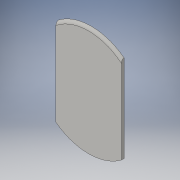
# Autodesk Inventor part: Nathan_RobotArm_Base
Saved by Autodesk Inventor 2016 (Build 200138000, 138)
## iProperties
Created: 2017-03-30
Part Number: Nathan_RobotArm_Base
Material: Generic
Document SubType Name: Modeling
Designer: brandn
Density: 1 g/cm^3
Appearance: Default
Author: brandn
Autodesk Inventor part; units mm, degrees
ref_plane "YZ Plane" through (0, 0, 0) normal (1, 0, 0) x (0, 1, 0)
ref_plane "XZ Plane" through (0, 0, 0) normal (0, 1, 0) x (-1, 0, 0)
ref_plane "XY Plane" through (0, 0, 0) normal (0, 0, 1) x (1, 0, 0)
sketch "Sketch1" plane through (0, 0, 0) normal (0, 0, 1) x (1, 0, 0)
  line L0 (-76.2, 12.7) -> (-76.2, 114.3)
  line L1 (0, 114.3) -> (0, 12.7)
  arc A0 (0, 114.3) -> (-76.2, 114.3) centre (-38.1, 63.5) ccw
  arc A1 (-76.2, 12.7) -> (0, 12.7) centre (-38.1, 63.5) ccw
  circle A2 centre (-38.1, 45.4023) radius 19.2368
  point P0 (0, 0)
  constraints: 4 end point, 4 point on circle, 3 centre point, 1 coincident, 1 parallel
extrude "Extrusion1" add sketch "Sketch1" along normal blind 3.175 contours L0 A0 L1 A1 | A2
fillet "Fillet1" radius 3.175 1 edges at (-38.1, 127, 3.175)
body "Solid1"
